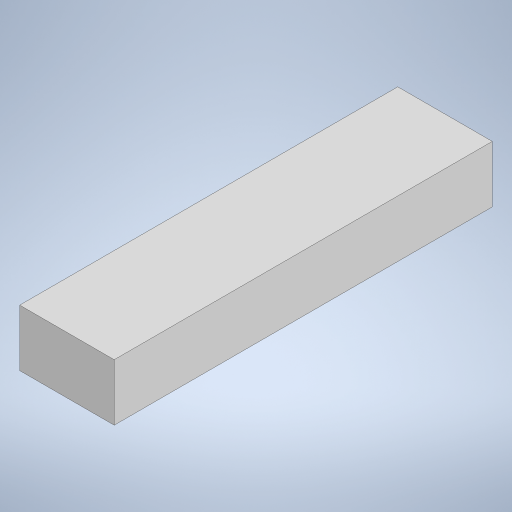
# Autodesk Inventor part: connect
Saved by Autodesk Inventor 2023 (Build 270158000, 158)
## iProperties
Created: 2024-06-09
Part Number: connect
Material: 常规
Document SubType Name: Modeling
Designer: Nitrene.P.L
Density: 1 g/cm^3
Appearance: 默认
Author: Nitrene.P.L
Autodesk Inventor part; units mm, degrees
ref_plane "YZ Plane" through (0, 0, 0) normal (1, 0, 0) x (0, 1, 0)
ref_plane "XZ Plane" through (0, 0, 0) normal (0, 1, 0) x (-1, 0, 0)
ref_plane "XY Plane" through (0, 0, 0) normal (0, 0, 1) x (1, 0, 0)
sketch "草图1" plane through (0, 0, 0) normal (0, 1, 0) x (-1, 0, 0)
  line L0 (5, 20) -> (-5, 20)
  line L1 (-5, 20) -> (-5, -20)
  line L2 (-5, -20) -> (5, -20)
  line L3 (5, -20) -> (5, 20)
  line L4 (0, 2.1988) -> (0, -1.8948)
  line L5 (1.3565, 0) -> (-1, 0)
  point P0 (0, 0)
  dimension "d0" = 10
  dimension "d1" = 40
  constraints: 12 end point, 2 horizontal, 2 parallel, 2 vertical, 1 perpendicular, 2 other
  measures "d0" distance of L2.end L1.end
  measures "d1" distance of L1.end L0.end
extrude "拉伸1" add sketch "草图1" along normal blind 6
